Autodesk Fusion 360 part; units mm, degrees
note: some values were not read from the file. Chosen so that the rebuilt part matches the saved one: which bodies a step acts on.
(part 4 of 5)
sketch "スケッチ1 (16)" plane through (0, 0, 0) normal (0, 0, 1) x (1, 0, 0) in component "Stage2_Planet_Gear_C"
  line L0 (-42.7218, 3.2284) -> (-43.6623, 3.4671)
  line L1 (-43.6623, 3.4671) -> (-44.4838, 3.4839)
  line L2 (-44.4838, 3.4839) -> (-45.3401, 3.3351)
  line L3 (-45.3401, 3.3351) -> (-46.2134, 3.0621)
  line L4 (-46.2134, 3.0621) -> (-46.3661, 2.098)
  line L5 (-46.3661, 2.098) -> (-45.6199, 1.5685)
  line L6 (-45.6199, 1.5685) -> (-44.8515, 1.1623)
  line L7 (-44.8515, 1.1623) -> (-44.065, 0.9245)
  line L8 (-44.065, 0.9245) -> (-43.0967, 0.8608)
  line L9 (-43.0967, 0.8608) -> (-43.125, 0)
  line L10 (-43.125, 0) -> (-43.0967, -0.8608)
  line L11 (-43.0967, -0.8608) -> (-44.065, -0.9245)
  line L12 (-44.065, -0.9245) -> (-44.8515, -1.1623)
  line L13 (-44.8515, -1.1623) -> (-45.6199, -1.5685)
  line L14 (-45.6199, -1.5685) -> (-46.3661, -2.098)
  line L15 (-46.3661, -2.098) -> (-46.2134, -3.0621)
  line L16 (-46.2134, -3.0621) -> (-45.3401, -3.3351)
  line L17 (-45.3401, -3.3351) -> (-44.4838, -3.4839)
  line L18 (-44.4838, -3.4839) -> (-43.6623, -3.4671)
  line L19 (-43.6623, -3.4671) -> (-42.7218, -3.2284)
  line L20 (-42.7218, -3.2284) -> (-42.4826, -4.0558)
  line L21 (-42.4826, -4.0558) -> (-42.1897, -4.8658)
  line L22 (-42.1897, -4.8658) -> (-43.091, -5.2256)
  line L23 (-43.091, -5.2256) -> (-43.7654, -5.6948)
  line L24 (-43.7654, -5.6948) -> (-44.3707, -6.3185)
  line L25 (-44.3707, -6.3185) -> (-44.9168, -7.0527)
  line L26 (-44.9168, -7.0527) -> (-44.4736, -7.9225)
  line L27 (-44.4736, -7.9225) -> (-43.5587, -7.9123)
  line L28 (-43.5587, -7.9123) -> (-42.6983, -7.7891)
  line L29 (-42.6983, -7.7891) -> (-41.9223, -7.5193)
  line L30 (-41.9223, -7.5193) -> (-41.1015, -7.0016)
  line L31 (-41.1015, -7.0016) -> (-40.6183, -7.7147)
  line L32 (-40.6183, -7.7147) -> (-40.0895, -8.3945)
  line L33 (-40.0895, -8.3945) -> (-40.8355, -9.0152)
  line L34 (-40.8355, -9.0152) -> (-41.3319, -9.6699)
  line L35 (-41.3319, -9.6699) -> (-41.7149, -10.4501)
  line L36 (-41.7149, -10.4501) -> (-42.0073, -11.317)
  line L37 (-42.0073, -11.317) -> (-41.317, -12.0073)
  line L38 (-41.317, -12.0073) -> (-40.4501, -11.7149)
  line L39 (-40.4501, -11.7149) -> (-39.6699, -11.3319)
  line L40 (-39.6699, -11.3319) -> (-39.0152, -10.8355)
  line L41 (-39.0152, -10.8355) -> (-38.3945, -10.0895)
  line L42 (-38.3945, -10.0895) -> (-37.7147, -10.6183)
  line L43 (-37.7147, -10.6183) -> (-37.0016, -11.1015)
  line L44 (-37.0016, -11.1015) -> (-37.5193, -11.9223)
  line L45 (-37.5193, -11.9223) -> (-37.7891, -12.6983)
  line L46 (-37.7891, -12.6983) -> (-37.9123, -13.5587)
  line L47 (-37.9123, -13.5587) -> (-37.9225, -14.4736)
  line L48 (-37.9225, -14.4736) -> (-37.0527, -14.9168)
  line L49 (-37.0527, -14.9168) -> (-36.3185, -14.3707)
  line L50 (-36.3185, -14.3707) -> (-35.6948, -13.7654)
  line L51 (-35.6948, -13.7654) -> (-35.2256, -13.091)
  line L52 (-35.2256, -13.091) -> (-34.8658, -12.1897)
  line L53 (-34.8658, -12.1897) -> (-34.0558, -12.4826)
  line L54 (-34.0558, -12.4826) -> (-33.2284, -12.7218)
  line L55 (-33.2284, -12.7218) -> (-33.4671, -13.6623)
  line L56 (-33.4671, -13.6623) -> (-33.4839, -14.4838)
  line L57 (-33.4839, -14.4838) -> (-33.3351, -15.3401)
  line L58 (-33.3351, -15.3401) -> (-33.0621, -16.2134)
  line L59 (-33.0621, -16.2134) -> (-32.098, -16.3661)
  line L60 (-32.098, -16.3661) -> (-31.5685, -15.6199)
  line L61 (-31.5685, -15.6199) -> (-31.1623, -14.8515)
  line L62 (-31.1623, -14.8515) -> (-30.9245, -14.065)
  line L63 (-30.9245, -14.065) -> (-30.8608, -13.0967)
  line L64 (-30.8608, -13.0967) -> (-30, -13.125)
  line L65 (-30, -13.125) -> (-29.1392, -13.0967)
  line L66 (-29.1392, -13.0967) -> (-29.0755, -14.065)
  line L67 (-29.0755, -14.065) -> (-28.8377, -14.8515)
  line L68 (-28.8377, -14.8515) -> (-28.4315, -15.6199)
  line L69 (-28.4315, -15.6199) -> (-27.902, -16.3661)
  line L70 (-27.902, -16.3661) -> (-26.9379, -16.2134)
  line L71 (-26.9379, -16.2134) -> (-26.6649, -15.3401)
  line L72 (-26.6649, -15.3401) -> (-26.5161, -14.4838)
  line L73 (-26.5161, -14.4838) -> (-26.5329, -13.6623)
  line L74 (-26.5329, -13.6623) -> (-26.7716, -12.7218)
  line L75 (-26.7716, -12.7218) -> (-25.9442, -12.4826)
  line L76 (-25.9442, -12.4826) -> (-25.1342, -12.1897)
  line L77 (-25.1342, -12.1897) -> (-24.7744, -13.091)
  line L78 (-24.7744, -13.091) -> (-24.3052, -13.7654)
  line L79 (-24.3052, -13.7654) -> (-23.6815, -14.3707)
  line L80 (-23.6815, -14.3707) -> (-22.9473, -14.9168)
  line L81 (-22.9473, -14.9168) -> (-22.0775, -14.4736)
  line L82 (-22.0775, -14.4736) -> (-22.0877, -13.5587)
  line L83 (-22.0877, -13.5587) -> (-22.2109, -12.6983)
  line L84 (-22.2109, -12.6983) -> (-22.4807, -11.9223)
  line L85 (-22.4807, -11.9223) -> (-22.9984, -11.1015)
  line L86 (-22.9984, -11.1015) -> (-22.2853, -10.6183)
  line L87 (-22.2853, -10.6183) -> (-21.6055, -10.0895)
  line L88 (-21.6055, -10.0895) -> (-20.9848, -10.8355)
  line L89 (-20.9848, -10.8355) -> (-20.3301, -11.3319)
  line L90 (-20.3301, -11.3319) -> (-19.5499, -11.7149)
  line L91 (-19.5499, -11.7149) -> (-18.683, -12.0073)
  line L92 (-18.683, -12.0073) -> (-17.9927, -11.317)
  line L93 (-17.9927, -11.317) -> (-18.2851, -10.4501)
  line L94 (-18.2851, -10.4501) -> (-18.6681, -9.6699)
  line L95 (-18.6681, -9.6699) -> (-19.1645, -9.0152)
  line L96 (-19.1645, -9.0152) -> (-19.9105, -8.3945)
  line L97 (-19.9105, -8.3945) -> (-19.3817, -7.7147)
  line L98 (-19.3817, -7.7147) -> (-18.8985, -7.0016)
  line L99 (-18.8985, -7.0016) -> (-18.0777, -7.5193)
  line L100 (-18.0777, -7.5193) -> (-17.3017, -7.7891)
  line L101 (-17.3017, -7.7891) -> (-16.4413, -7.9123)
  line L102 (-16.4413, -7.9123) -> (-15.5264, -7.9225)
  line L103 (-15.5264, -7.9225) -> (-15.0832, -7.0527)
  line L104 (-15.0832, -7.0527) -> (-15.6293, -6.3185)
  line L105 (-15.6293, -6.3185) -> (-16.2346, -5.6948)
  line L106 (-16.2346, -5.6948) -> (-16.909, -5.2256)
  line L107 (-16.909, -5.2256) -> (-17.8103, -4.8658)
  line L108 (-17.8103, -4.8658) -> (-17.5174, -4.0558)
  line L109 (-17.5174, -4.0558) -> (-17.2782, -3.2284)
  line L110 (-17.2782, -3.2284) -> (-16.3377, -3.4671)
  line L111 (-16.3377, -3.4671) -> (-15.5162, -3.4839)
  line L112 (-15.5162, -3.4839) -> (-14.6599, -3.3351)
  line L113 (-14.6599, -3.3351) -> (-13.7866, -3.0621)
  line L114 (-13.7866, -3.0621) -> (-13.6339, -2.098)
  line L115 (-13.6339, -2.098) -> (-14.3801, -1.5685)
  line L116 (-14.3801, -1.5685) -> (-15.1485, -1.1623)
  line L117 (-15.1485, -1.1623) -> (-15.935, -0.9245)
  line L118 (-15.935, -0.9245) -> (-16.9033, -0.8608)
  line L119 (-16.9033, -0.8608) -> (-16.875, 0)
  line L120 (-16.875, 0) -> (-16.9033, 0.8608)
  line L121 (-16.9033, 0.8608) -> (-15.935, 0.9245)
  line L122 (-15.935, 0.9245) -> (-15.1485, 1.1623)
  line L123 (-15.1485, 1.1623) -> (-14.3801, 1.5685)
  line L124 (-14.3801, 1.5685) -> (-13.6339, 2.098)
  line L125 (-13.6339, 2.098) -> (-13.7866, 3.0621)
  line L126 (-13.7866, 3.0621) -> (-14.6599, 3.3351)
  line L127 (-14.6599, 3.3351) -> (-15.5162, 3.4839)
  line L128 (-15.5162, 3.4839) -> (-16.3377, 3.4671)
  line L129 (-16.3377, 3.4671) -> (-17.2782, 3.2284)
  line L130 (-17.2782, 3.2284) -> (-17.5174, 4.0558)
  line L131 (-17.5174, 4.0558) -> (-17.8103, 4.8658)
  line L132 (-17.8103, 4.8658) -> (-16.909, 5.2256)
  line L133 (-16.909, 5.2256) -> (-16.2346, 5.6948)
  line L134 (-16.2346, 5.6948) -> (-15.6293, 6.3185)
  line L135 (-15.6293, 6.3185) -> (-15.0832, 7.0527)
  line L136 (-15.0832, 7.0527) -> (-15.5264, 7.9225)
  line L137 (-15.5264, 7.9225) -> (-16.4413, 7.9123)
  line L138 (-16.4413, 7.9123) -> (-17.3017, 7.7891)
  line L139 (-17.3017, 7.7891) -> (-18.0777, 7.5193)
  line L140 (-18.0777, 7.5193) -> (-18.8985, 7.0016)
  line L141 (-18.8985, 7.0016) -> (-19.3817, 7.7147)
  line L142 (-19.3817, 7.7147) -> (-19.9105, 8.3945)
  line L143 (-19.9105, 8.3945) -> (-19.1645, 9.0152)
  line L144 (-19.1645, 9.0152) -> (-18.6681, 9.6699)
  line L145 (-18.6681, 9.6699) -> (-18.2851, 10.4501)
  line L146 (-18.2851, 10.4501) -> (-17.9927, 11.317)
  line L147 (-17.9927, 11.317) -> (-18.683, 12.0073)
  line L148 (-18.683, 12.0073) -> (-19.5499, 11.7149)
  line L149 (-19.5499, 11.7149) -> (-20.3301, 11.3319)
  line L150 (-20.3301, 11.3319) -> (-20.9848, 10.8355)
  line L151 (-20.9848, 10.8355) -> (-21.6055, 10.0895)
  line L152 (-21.6055, 10.0895) -> (-22.2853, 10.6183)
  line L153 (-22.2853, 10.6183) -> (-22.9984, 11.1015)
  line L154 (-22.9984, 11.1015) -> (-22.4807, 11.9223)
  line L155 (-22.4807, 11.9223) -> (-22.2109, 12.6983)
  line L156 (-22.2109, 12.6983) -> (-22.0877, 13.5587)
  line L157 (-22.0877, 13.5587) -> (-22.0775, 14.4736)
  line L158 (-22.0775, 14.4736) -> (-22.9473, 14.9168)
  line L159 (-22.9473, 14.9168) -> (-23.6815, 14.3707)
  line L160 (-23.6815, 14.3707) -> (-24.3052, 13.7654)
  line L161 (-24.3052, 13.7654) -> (-24.7744, 13.091)
  line L162 (-24.7744, 13.091) -> (-25.1342, 12.1897)
  line L163 (-25.1342, 12.1897) -> (-25.9442, 12.4826)
  line L164 (-25.9442, 12.4826) -> (-26.7716, 12.7218)
  line L165 (-26.7716, 12.7218) -> (-26.5329, 13.6623)
  line L166 (-26.5329, 13.6623) -> (-26.5161, 14.4838)
  line L167 (-26.5161, 14.4838) -> (-26.6649, 15.3401)
  line L168 (-26.6649, 15.3401) -> (-26.9379, 16.2134)
  line L169 (-26.9379, 16.2134) -> (-27.902, 16.3661)
  line L170 (-27.902, 16.3661) -> (-28.4315, 15.6199)
  line L171 (-28.4315, 15.6199) -> (-28.8377, 14.8515)
  line L172 (-28.8377, 14.8515) -> (-29.0755, 14.065)
  line L173 (-29.0755, 14.065) -> (-29.1392, 13.0967)
  line L174 (-29.1392, 13.0967) -> (-30, 13.125)
  line L175 (-30, 13.125) -> (-30.8608, 13.0967)
  line L176 (-30.8608, 13.0967) -> (-30.9245, 14.065)
  line L177 (-30.9245, 14.065) -> (-31.1623, 14.8515)
  line L178 (-31.1623, 14.8515) -> (-31.5685, 15.6199)
  line L179 (-31.5685, 15.6199) -> (-32.098, 16.3661)
  line L180 (-32.098, 16.3661) -> (-33.0621, 16.2134)
  line L181 (-33.0621, 16.2134) -> (-33.3351, 15.3401)
  line L182 (-33.3351, 15.3401) -> (-33.4839, 14.4838)
  line L183 (-33.4839, 14.4838) -> (-33.4671, 13.6623)
  line L184 (-33.4671, 13.6623) -> (-33.2284, 12.7218)
  line L185 (-33.2284, 12.7218) -> (-34.0558, 12.4826)
  line L186 (-34.0558, 12.4826) -> (-34.8658, 12.1897)
  line L187 (-34.8658, 12.1897) -> (-35.2256, 13.091)
  line L188 (-35.2256, 13.091) -> (-35.6948, 13.7654)
  line L189 (-35.6948, 13.7654) -> (-36.3185, 14.3707)
  line L190 (-36.3185, 14.3707) -> (-37.0527, 14.9168)
  line L191 (-37.0527, 14.9168) -> (-37.9225, 14.4736)
  line L192 (-37.9225, 14.4736) -> (-37.9123, 13.5587)
  line L193 (-37.9123, 13.5587) -> (-37.7891, 12.6983)
  line L194 (-37.7891, 12.6983) -> (-37.5193, 11.9223)
  line L195 (-37.5193, 11.9223) -> (-37.0016, 11.1015)
  line L196 (-37.0016, 11.1015) -> (-37.7147, 10.6183)
  line L197 (-37.7147, 10.6183) -> (-38.3945, 10.0895)
  line L198 (-38.3945, 10.0895) -> (-39.0152, 10.8355)
  line L199 (-39.0152, 10.8355) -> (-39.6699, 11.3319)
  line L200 (-39.6699, 11.3319) -> (-40.4501, 11.7149)
  line L201 (-40.4501, 11.7149) -> (-41.317, 12.0073)
  line L202 (-41.317, 12.0073) -> (-42.0073, 11.317)
  line L203 (-42.0073, 11.317) -> (-41.7149, 10.4501)
  line L204 (-41.7149, 10.4501) -> (-41.3319, 9.6699)
  line L205 (-41.3319, 9.6699) -> (-40.8355, 9.0152)
  line L206 (-40.8355, 9.0152) -> (-40.0895, 8.3945)
  line L207 (-40.0895, 8.3945) -> (-40.6183, 7.7147)
  line L208 (-40.6183, 7.7147) -> (-41.1015, 7.0016)
  line L209 (-41.1015, 7.0016) -> (-41.9223, 7.5193)
  line L210 (-41.9223, 7.5193) -> (-42.6983, 7.7891)
  line L211 (-42.6983, 7.7891) -> (-43.5587, 7.9123)
  line L212 (-43.5587, 7.9123) -> (-44.4736, 7.9225)
  line L213 (-44.4736, 7.9225) -> (-44.9168, 7.0527)
  line L214 (-44.9168, 7.0527) -> (-44.3707, 6.3185)
  line L215 (-44.3707, 6.3185) -> (-43.7654, 5.6948)
  line L216 (-43.7654, 5.6948) -> (-43.091, 5.2256)
  line L217 (-43.091, 5.2256) -> (-42.1897, 4.8658)
  line L218 (-42.1897, 4.8658) -> (-42.4826, 4.0558)
  line L219 (-42.4826, 4.0558) -> (-42.7218, 3.2284)
extrude "Stage2_Planet_C_Extrude" add sketch "スケッチ1 (16)" along normal blind 12 from surface at 74 separate body makes body 17 in component "Stage2_Planet_Gear_C"
sketch "スケッチ2 (16)" plane through (0, 0, 0) normal (0, 0, 1) x (1, 0, 0) in component "Stage2_Planet_Gear_C"
  circle A0 centre (-30, 0) radius 9
extrude "Stage2_Planet_C_Hub_Lower_Extrude" add sketch "スケッチ2 (16)" along normal blind 3 from surface at 71 bodies 17 in component "Stage2_Planet_Gear_C"
sketch "スケッチ3 (15)" plane through (0, 0, 0) normal (0, 0, 1) x (1, 0, 0) in component "Stage2_Planet_Gear_C"
  circle A0 centre (-30, 0) radius 9
extrude "Stage2_Planet_C_Hub_Upper_Extrude" add sketch "スケッチ3 (15)" along normal blind 3 from surface at 86 bodies 17 in component "Stage2_Planet_Gear_C"
sketch "スケッチ4 (15)" plane through (0, 0, 0) normal (0, 0, 1) x (1, 0, 0) in component "Stage2_Planet_Gear_C"
  circle A0 centre (-30, 0) radius 4.3
extrude "Stage2_Planet_C_Bore_Cut" cut sketch "スケッチ4 (15)" along normal blind 20 from surface at 70 bodies 17 in component "Stage2_Planet_Gear_C"
sketch "スケッチ1 (17)" plane through (0, 0, 0) normal (0, 0, 1) x (1, 0, 0) in component "Stage2_Planet_Gear_D"
  line L0 (-12.7218, -26.7716) -> (-13.6623, -26.5329)
  line L1 (-13.6623, -26.5329) -> (-14.4838, -26.5161)
  line L2 (-14.4838, -26.5161) -> (-15.3401, -26.6649)
  line L3 (-15.3401, -26.6649) -> (-16.2134, -26.9379)
  line L4 (-16.2134, -26.9379) -> (-16.3661, -27.902)
  line L5 (-16.3661, -27.902) -> (-15.6199, -28.4315)
  line L6 (-15.6199, -28.4315) -> (-14.8515, -28.8377)
  line L7 (-14.8515, -28.8377) -> (-14.065, -29.0755)
  line L8 (-14.065, -29.0755) -> (-13.0967, -29.1392)
  line L9 (-13.0967, -29.1392) -> (-13.125, -30)
  line L10 (-13.125, -30) -> (-13.0967, -30.8608)
  line L11 (-13.0967, -30.8608) -> (-14.065, -30.9245)
  line L12 (-14.065, -30.9245) -> (-14.8515, -31.1623)
  line L13 (-14.8515, -31.1623) -> (-15.6199, -31.5685)
  line L14 (-15.6199, -31.5685) -> (-16.3661, -32.098)
  line L15 (-16.3661, -32.098) -> (-16.2134, -33.0621)
  line L16 (-16.2134, -33.0621) -> (-15.3401, -33.3351)
  line L17 (-15.3401, -33.3351) -> (-14.4838, -33.4839)
  line L18 (-14.4838, -33.4839) -> (-13.6623, -33.4671)
  line L19 (-13.6623, -33.4671) -> (-12.7218, -33.2284)
  line L20 (-12.7218, -33.2284) -> (-12.4826, -34.0558)
  line L21 (-12.4826, -34.0558) -> (-12.1897, -34.8658)
  line L22 (-12.1897, -34.8658) -> (-13.091, -35.2256)
  line L23 (-13.091, -35.2256) -> (-13.7654, -35.6948)
  line L24 (-13.7654, -35.6948) -> (-14.3707, -36.3185)
  line L25 (-14.3707, -36.3185) -> (-14.9168, -37.0527)
  line L26 (-14.9168, -37.0527) -> (-14.4736, -37.9225)
  line L27 (-14.4736, -37.9225) -> (-13.5587, -37.9123)
  line L28 (-13.5587, -37.9123) -> (-12.6983, -37.7891)
  line L29 (-12.6983, -37.7891) -> (-11.9223, -37.5193)
  line L30 (-11.9223, -37.5193) -> (-11.1015, -37.0016)
  line L31 (-11.1015, -37.0016) -> (-10.6183, -37.7147)
  line L32 (-10.6183, -37.7147) -> (-10.0895, -38.3945)
  line L33 (-10.0895, -38.3945) -> (-10.8355, -39.0152)
  line L34 (-10.8355, -39.0152) -> (-11.3319, -39.6699)
  line L35 (-11.3319, -39.6699) -> (-11.7149, -40.4501)
  line L36 (-11.7149, -40.4501) -> (-12.0073, -41.317)
  line L37 (-12.0073, -41.317) -> (-11.317, -42.0073)
  line L38 (-11.317, -42.0073) -> (-10.4501, -41.7149)
  line L39 (-10.4501, -41.7149) -> (-9.6699, -41.3319)
  line L40 (-9.6699, -41.3319) -> (-9.0152, -40.8355)
  line L41 (-9.0152, -40.8355) -> (-8.3945, -40.0895)
  line L42 (-8.3945, -40.0895) -> (-7.7147, -40.6183)
  line L43 (-7.7147, -40.6183) -> (-7.0016, -41.1015)
  line L44 (-7.0016, -41.1015) -> (-7.5193, -41.9223)
  line L45 (-7.5193, -41.9223) -> (-7.7891, -42.6983)
  line L46 (-7.7891, -42.6983) -> (-7.9123, -43.5587)
  line L47 (-7.9123, -43.5587) -> (-7.9225, -44.4736)
  line L48 (-7.9225, -44.4736) -> (-7.0527, -44.9168)
  line L49 (-7.0527, -44.9168) -> (-6.3185, -44.3707)
  line L50 (-6.3185, -44.3707) -> (-5.6948, -43.7654)
  line L51 (-5.6948, -43.7654) -> (-5.2256, -43.091)
  line L52 (-5.2256, -43.091) -> (-4.8658, -42.1897)
  line L53 (-4.8658, -42.1897) -> (-4.0558, -42.4826)
  line L54 (-4.0558, -42.4826) -> (-3.2284, -42.7218)
  line L55 (-3.2284, -42.7218) -> (-3.4671, -43.6623)
  line L56 (-3.4671, -43.6623) -> (-3.4839, -44.4838)
  line L57 (-3.4839, -44.4838) -> (-3.3351, -45.3401)
  line L58 (-3.3351, -45.3401) -> (-3.0621, -46.2134)
  line L59 (-3.0621, -46.2134) -> (-2.098, -46.3661)
  line L60 (-2.098, -46.3661) -> (-1.5685, -45.6199)
  line L61 (-1.5685, -45.6199) -> (-1.1623, -44.8515)
  line L62 (-1.1623, -44.8515) -> (-0.9245, -44.065)
  line L63 (-0.9245, -44.065) -> (-0.8608, -43.0967)
  line L64 (-0.8608, -43.0967) -> (0, -43.125)
  line L65 (0, -43.125) -> (0.8608, -43.0967)
  line L66 (0.8608, -43.0967) -> (0.9245, -44.065)
  line L67 (0.9245, -44.065) -> (1.1623, -44.8515)
  line L68 (1.1623, -44.8515) -> (1.5685, -45.6199)
  line L69 (1.5685, -45.6199) -> (2.098, -46.3661)
  line L70 (2.098, -46.3661) -> (3.0621, -46.2134)
  line L71 (3.0621, -46.2134) -> (3.3351, -45.3401)
  line L72 (3.3351, -45.3401) -> (3.4839, -44.4838)
  line L73 (3.4839, -44.4838) -> (3.4671, -43.6623)
  line L74 (3.4671, -43.6623) -> (3.2284, -42.7218)
  line L75 (3.2284, -42.7218) -> (4.0558, -42.4826)
  line L76 (4.0558, -42.4826) -> (4.8658, -42.1897)
  line L77 (4.8658, -42.1897) -> (5.2256, -43.091)
  line L78 (5.2256, -43.091) -> (5.6948, -43.7654)
  line L79 (5.6948, -43.7654) -> (6.3185, -44.3707)
  line L80 (6.3185, -44.3707) -> (7.0527, -44.9168)
  line L81 (7.0527, -44.9168) -> (7.9225, -44.4736)
  line L82 (7.9225, -44.4736) -> (7.9123, -43.5587)
  line L83 (7.9123, -43.5587) -> (7.7891, -42.6983)
  line L84 (7.7891, -42.6983) -> (7.5193, -41.9223)
  line L85 (7.5193, -41.9223) -> (7.0016, -41.1015)
  line L86 (7.0016, -41.1015) -> (7.7147, -40.6183)
  line L87 (7.7147, -40.6183) -> (8.3945, -40.0895)
  line L88 (8.3945, -40.0895) -> (9.0152, -40.8355)
  line L89 (9.0152, -40.8355) -> (9.6699, -41.3319)
  line L90 (9.6699, -41.3319) -> (10.4501, -41.7149)
  line L91 (10.4501, -41.7149) -> (11.317, -42.0073)
  line L92 (11.317, -42.0073) -> (12.0073, -41.317)
  line L93 (12.0073, -41.317) -> (11.7149, -40.4501)
  line L94 (11.7149, -40.4501) -> (11.3319, -39.6699)
  line L95 (11.3319, -39.6699) -> (10.8355, -39.0152)
  line L96 (10.8355, -39.0152) -> (10.0895, -38.3945)
  line L97 (10.0895, -38.3945) -> (10.6183, -37.7147)
  line L98 (10.6183, -37.7147) -> (11.1015, -37.0016)
  line L99 (11.1015, -37.0016) -> (11.9223, -37.5193)
  line L100 (11.9223, -37.5193) -> (12.6983, -37.7891)
  line L101 (12.6983, -37.7891) -> (13.5587, -37.9123)
  line L102 (13.5587, -37.9123) -> (14.4736, -37.9225)
  line L103 (14.4736, -37.9225) -> (14.9168, -37.0527)
  line L104 (14.9168, -37.0527) -> (14.3707, -36.3185)
  line L105 (14.3707, -36.3185) -> (13.7654, -35.6948)
  line L106 (13.7654, -35.6948) -> (13.091, -35.2256)
  line L107 (13.091, -35.2256) -> (12.1897, -34.8658)
  line L108 (12.1897, -34.8658) -> (12.4826, -34.0558)
  line L109 (12.4826, -34.0558) -> (12.7218, -33.2284)
  line L110 (12.7218, -33.2284) -> (13.6623, -33.4671)
  line L111 (13.6623, -33.4671) -> (14.4838, -33.4839)
  line L112 (14.4838, -33.4839) -> (15.3401, -33.3351)
  line L113 (15.3401, -33.3351) -> (16.2134, -33.0621)
  line L114 (16.2134, -33.0621) -> (16.3661, -32.098)
  line L115 (16.3661, -32.098) -> (15.6199, -31.5685)
  line L116 (15.6199, -31.5685) -> (14.8515, -31.1623)
  line L117 (14.8515, -31.1623) -> (14.065, -30.9245)
  line L118 (14.065, -30.9245) -> (13.0967, -30.8608)
  line L119 (13.0967, -30.8608) -> (13.125, -30)
  line L120 (13.125, -30) -> (13.0967, -29.1392)
  line L121 (13.0967, -29.1392) -> (14.065, -29.0755)
  line L122 (14.065, -29.0755) -> (14.8515, -28.8377)
  line L123 (14.8515, -28.8377) -> (15.6199, -28.4315)
  line L124 (15.6199, -28.4315) -> (16.3661, -27.902)
  line L125 (16.3661, -27.902) -> (16.2134, -26.9379)
  line L126 (16.2134, -26.9379) -> (15.3401, -26.6649)
  line L127 (15.3401, -26.6649) -> (14.4838, -26.5161)
  line L128 (14.4838, -26.5161) -> (13.6623, -26.5329)
  line L129 (13.6623, -26.5329) -> (12.7218, -26.7716)
  line L130 (12.7218, -26.7716) -> (12.4826, -25.9442)
  line L131 (12.4826, -25.9442) -> (12.1897, -25.1342)
  line L132 (12.1897, -25.1342) -> (13.091, -24.7744)
  line L133 (13.091, -24.7744) -> (13.7654, -24.3052)
  line L134 (13.7654, -24.3052) -> (14.3707, -23.6815)
  line L135 (14.3707, -23.6815) -> (14.9168, -22.9473)
  line L136 (14.9168, -22.9473) -> (14.4736, -22.0775)
  line L137 (14.4736, -22.0775) -> (13.5587, -22.0877)
  line L138 (13.5587, -22.0877) -> (12.6983, -22.2109)
  line L139 (12.6983, -22.2109) -> (11.9223, -22.4807)
  line L140 (11.9223, -22.4807) -> (11.1015, -22.9984)
  line L141 (11.1015, -22.9984) -> (10.6183, -22.2853)
  line L142 (10.6183, -22.2853) -> (10.0895, -21.6055)
  line L143 (10.0895, -21.6055) -> (10.8355, -20.9848)
  line L144 (10.8355, -20.9848) -> (11.3319, -20.3301)
  line L145 (11.3319, -20.3301) -> (11.7149, -19.5499)
  line L146 (11.7149, -19.5499) -> (12.0073, -18.683)
  line L147 (12.0073, -18.683) -> (11.317, -17.9927)
  line L148 (11.317, -17.9927) -> (10.4501, -18.2851)
  line L149 (10.4501, -18.2851) -> (9.6699, -18.6681)
  line L150 (9.6699, -18.6681) -> (9.0152, -19.1645)
  line L151 (9.0152, -19.1645) -> (8.3945, -19.9105)
  line L152 (8.3945, -19.9105) -> (7.7147, -19.3817)
  line L153 (7.7147, -19.3817) -> (7.0016, -18.8985)
  line L154 (7.0016, -18.8985) -> (7.5193, -18.0777)
  line L155 (7.5193, -18.0777) -> (7.7891, -17.3017)
  line L156 (7.7891, -17.3017) -> (7.9123, -16.4413)
  line L157 (7.9123, -16.4413) -> (7.9225, -15.5264)
  line L158 (7.9225, -15.5264) -> (7.0527, -15.0832)
  line L159 (7.0527, -15.0832) -> (6.3185, -15.6293)
  line L160 (6.3185, -15.6293) -> (5.6948, -16.2346)
  line L161 (5.6948, -16.2346) -> (5.2256, -16.909)
  line L162 (5.2256, -16.909) -> (4.8658, -17.8103)
  line L163 (4.8658, -17.8103) -> (4.0558, -17.5174)
  line L164 (4.0558, -17.5174) -> (3.2284, -17.2782)
  line L165 (3.2284, -17.2782) -> (3.4671, -16.3377)
  line L166 (3.4671, -16.3377) -> (3.4839, -15.5162)
  line L167 (3.4839, -15.5162) -> (3.3351, -14.6599)
  line L168 (3.3351, -14.6599) -> (3.0621, -13.7866)
  line L169 (3.0621, -13.7866) -> (2.098, -13.6339)
  line L170 (2.098, -13.6339) -> (1.5685, -14.3801)
  line L171 (1.5685, -14.3801) -> (1.1623, -15.1485)
  line L172 (1.1623, -15.1485) -> (0.9245, -15.935)
  line L173 (0.9245, -15.935) -> (0.8608, -16.9033)
  line L174 (0.8608, -16.9033) -> (0, -16.875)
  line L175 (0, -16.875) -> (-0.8608, -16.9033)
  line L176 (-0.8608, -16.9033) -> (-0.9245, -15.935)
  line L177 (-0.9245, -15.935) -> (-1.1623, -15.1485)
  line L178 (-1.1623, -15.1485) -> (-1.5685, -14.3801)
  line L179 (-1.5685, -14.3801) -> (-2.098, -13.6339)
  line L180 (-2.098, -13.6339) -> (-3.0621, -13.7866)
  line L181 (-3.0621, -13.7866) -> (-3.3351, -14.6599)
  line L182 (-3.3351, -14.6599) -> (-3.4839, -15.5162)
  line L183 (-3.4839, -15.5162) -> (-3.4671, -16.3377)
  line L184 (-3.4671, -16.3377) -> (-3.2284, -17.2782)
  line L185 (-3.2284, -17.2782) -> (-4.0558, -17.5174)
  line L186 (-4.0558, -17.5174) -> (-4.8658, -17.8103)
  line L187 (-4.8658, -17.8103) -> (-5.2256, -16.909)
  line L188 (-5.2256, -16.909) -> (-5.6948, -16.2346)
  line L189 (-5.6948, -16.2346) -> (-6.3185, -15.6293)
  line L190 (-6.3185, -15.6293) -> (-7.0527, -15.0832)
  line L191 (-7.0527, -15.0832) -> (-7.9225, -15.5264)
  line L192 (-7.9225, -15.5264) -> (-7.9123, -16.4413)
  line L193 (-7.9123, -16.4413) -> (-7.7891, -17.3017)
  line L194 (-7.7891, -17.3017) -> (-7.5193, -18.0777)
  line L195 (-7.5193, -18.0777) -> (-7.0016, -18.8985)
  line L196 (-7.0016, -18.8985) -> (-7.7147, -19.3817)
  line L197 (-7.7147, -19.3817) -> (-8.3945, -19.9105)
  line L198 (-8.3945, -19.9105) -> (-9.0152, -19.1645)
  line L199 (-9.0152, -19.1645) -> (-9.6699, -18.6681)
  line L200 (-9.6699, -18.6681) -> (-10.4501, -18.2851)
  line L201 (-10.4501, -18.2851) -> (-11.317, -17.9927)
  line L202 (-11.317, -17.9927) -> (-12.0073, -18.683)
  line L203 (-12.0073, -18.683) -> (-11.7149, -19.5499)
  line L204 (-11.7149, -19.5499) -> (-11.3319, -20.3301)
  line L205 (-11.3319, -20.3301) -> (-10.8355, -20.9848)
  line L206 (-10.8355, -20.9848) -> (-10.0895, -21.6055)
  line L207 (-10.0895, -21.6055) -> (-10.6183, -22.2853)
  line L208 (-10.6183, -22.2853) -> (-11.1015, -22.9984)
  line L209 (-11.1015, -22.9984) -> (-11.9223, -22.4807)
  line L210 (-11.9223, -22.4807) -> (-12.6983, -22.2109)
  line L211 (-12.6983, -22.2109) -> (-13.5587, -22.0877)
  line L212 (-13.5587, -22.0877) -> (-14.4736, -22.0775)
  line L213 (-14.4736, -22.0775) -> (-14.9168, -22.9473)
  line L214 (-14.9168, -22.9473) -> (-14.3707, -23.6815)
  line L215 (-14.3707, -23.6815) -> (-13.7654, -24.3052)
  line L216 (-13.7654, -24.3052) -> (-13.091, -24.7744)
  line L217 (-13.091, -24.7744) -> (-12.1897, -25.1342)
  line L218 (-12.1897, -25.1342) -> (-12.4826, -25.9442)
  line L219 (-12.4826, -25.9442) -> (-12.7218, -26.7716)
extrude "Stage2_Planet_D_Extrude" add sketch "スケッチ1 (17)" along normal blind 12 from surface at 74 separate body makes body 18 in component "Stage2_Planet_Gear_D"
sketch "スケッチ2 (17)" plane through (0, 0, 0) normal (0, 0, 1) x (1, 0, 0) in component "Stage2_Planet_Gear_D"
  circle A0 centre (0, -30) radius 9
extrude "Stage2_Planet_D_Hub_Lower_Extrude" add sketch "スケッチ2 (17)" along normal blind 3 from surface at 71 bodies 18 in component "Stage2_Planet_Gear_D"
sketch "スケッチ3 (16)" plane through (0, 0, 0) normal (0, 0, 1) x (1, 0, 0) in component "Stage2_Planet_Gear_D"
  circle A0 centre (0, -30) radius 9
extrude "Stage2_Planet_D_Hub_Upper_Extrude" add sketch "スケッチ3 (16)" along normal blind 3 from surface at 86 bodies 18 in component "Stage2_Planet_Gear_D"
sketch "スケッチ4 (16)" plane through (0, 0, 0) normal (0, 0, 1) x (1, 0, 0) in component "Stage2_Planet_Gear_D"
  circle A0 centre (0, -30) radius 4.3
extrude "Stage2_Planet_D_Bore_Cut" cut sketch "スケッチ4 (16)" along normal blind 20 from surface at 70 bodies 18 in component "Stage2_Planet_Gear_D"
sketch "スケッチ1 (18)" plane through (0, 0, 0) normal (0, 0, 1) x (1, 0, 0) in component "Stage2_Internal_Ring_Gear"
  circle A0 centre (0, 0) radius 58
extrude "Stage2_Ring_Extrude" add sketch "スケッチ1 (18)" along normal blind 12 from surface at 74 separate body makes body 19 in component "Stage2_Internal_Ring_Gear"
sketch "スケッチ2 (18)" plane through (0, 0, 0) normal (0, 0, 1) x (1, 0, 0) in component "Stage2_Internal_Ring_Gear"
  circle A0 centre (0, 0) radius 65.5
extrude "Stage2_Ring_Flange_Extrude" add sketch "スケッチ2 (18)" along normal blind 7 from surface at 76.5 bodies 19 in component "Stage2_Internal_Ring_Gear"
sketch "スケッチ3 (17)" plane through (0, 0, 0) normal (0, 0, 1) x (1, 0, 0) in component "Stage2_Internal_Ring_Gear"
  line L0 (46.8321, -2.0047) -> (45.171, -1.2223)
  line L1 (45.171, -1.2223) -> (43.495, -0.6584)
  line L2 (43.495, -0.6584) -> (43.495, 0.6584)
  line L3 (43.495, 0.6584) -> (45.171, 1.2223)
  line L4 (45.171, 1.2223) -> (46.8321, 2.0047)
  line L5 (46.8321, 2.0047) -> (46.8108, 2.4532)
  line L6 (46.8108, 2.4532) -> (46.7851, 2.9016)
  line L7 (46.7851, 2.9016) -> (45.0513, 3.506)
  line L8 (45.0513, 3.506) -> (43.3256, 3.8917)
  line L9 (43.3256, 3.8917) -> (43.1879, 5.2013)
  line L10 (43.1879, 5.2013) -> (44.7957, 5.9373)
  line L11 (44.7957, 5.9373) -> (46.366, 6.889)
  line L12 (46.366, 6.889) -> (46.2979, 7.3329)
  line L13 (46.2979, 7.3329) -> (46.2255, 7.7761)
  line L14 (46.2255, 7.7761) -> (44.438, 8.196)
  line L15 (44.438, 8.196) -> (42.6814, 8.3991)
  line L16 (42.6814, 8.3991) -> (42.4077, 9.6871)
  line L17 (42.4077, 9.6871) -> (43.9297, 10.5872)
  line L18 (43.9297, 10.5872) -> (45.3919, 11.6978)
  line L19 (45.3919, 11.6978) -> (45.2778, 12.1321)
  line L20 (45.2778, 12.1321) -> (45.1595, 12.5653)
  line L21 (45.1595, 12.5653) -> (43.3379, 12.7961)
  line L22 (43.3379, 12.7961) -> (41.5697, 12.8145)
  line L23 (41.5697, 12.8145) -> (41.1628, 14.0669)
  line L24 (41.1628, 14.0669) -> (42.5824, 15.1211)
  line L25 (42.5824, 15.1211) -> (43.9205, 16.3785)
  line L26 (43.9205, 16.3785) -> (43.7616, 16.7985)
  line L27 (43.7616, 16.7985) -> (43.5986, 17.217)
  line L28 (43.5986, 17.217) -> (41.7629, 17.256)
  line L29 (41.7629, 17.256) -> (40.0025, 17.0895)
  line L30 (40.0025, 17.0895) -> (39.4669, 18.2925)
  line L31 (39.4669, 18.2925) -> (40.7686, 19.4893)
  line L32 (40.7686, 19.4893) -> (41.9679, 20.8797)
  line L33 (41.9679, 20.8797) -> (41.7659, 21.2808)
  line L34 (41.7659, 21.2808) -> (41.5601, 21.6799)
  line L35 (41.5601, 21.6799) -> (39.7304, 21.5269)
  line L36 (39.7304, 21.5269) -> (37.997, 21.1773)
  line L37 (37.997, 21.1773) -> (37.3386, 22.3177)
  line L38 (37.3386, 22.3177) -> (38.508, 23.644)
  line L39 (38.508, 23.644) -> (39.5555, 25.1522)
  line L40 (39.5555, 25.1522) -> (39.3127, 25.53)
  line L41 (39.3127, 25.53) -> (39.0663, 25.9054)
  line L42 (39.0663, 25.9054) -> (37.2625, 25.5619)
  line L43 (37.2625, 25.5619) -> (35.5752, 25.0331)
  line L44 (35.5752, 25.0331) -> (34.8012, 26.0984)
  line L45 (34.8012, 26.0984) -> (35.8256, 27.5397)
  line L46 (35.8256, 27.5397) -> (36.7096, 29.1491)
  line L47 (36.7096, 29.1491) -> (36.4287, 29.4994)
  line L48 (36.4287, 29.4994) -> (36.1444, 29.847)
  line L49 (36.1444, 29.847) -> (34.3865, 29.3169)
  line L50 (34.3865, 29.3169) -> (32.7636, 28.6146)
  line L51 (32.7636, 28.6146) -> (31.8825, 29.5931)
  line L52 (31.8825, 29.5931) -> (32.7507, 31.1336)
  line L53 (32.7507, 31.1336) -> (33.4616, 32.8266)
  line L54 (33.4616, 32.8266) -> (33.1456, 33.1456)
  line L55 (33.1456, 33.1456) -> (32.8266, 33.4616)
  line L56 (32.8266, 33.4616) -> (31.1336, 32.7507)
  line L57 (31.1336, 32.7507) -> (29.5931, 31.8825)
  line L58 (29.5931, 31.8825) -> (28.6146, 32.7636)
  line L59 (28.6146, 32.7636) -> (29.3169, 34.3865)
  line L60 (29.3169, 34.3865) -> (29.847, 36.1444)
  line L61 (29.847, 36.1444) -> (29.4994, 36.4287)
  line L62 (29.4994, 36.4287) -> (29.1491, 36.7096)
  line L63 (29.1491, 36.7096) -> (27.5397, 35.8256)
  line L64 (27.5397, 35.8256) -> (26.0984, 34.8012)
  line L65 (26.0984, 34.8012) -> (25.0331, 35.5752)
  line L66 (25.0331, 35.5752) -> (25.5619, 37.2625)
  line L67 (25.5619, 37.2625) -> (25.9054, 39.0663)
  line L68 (25.9054, 39.0663) -> (25.53, 39.3127)
  line L69 (25.53, 39.3127) -> (25.1522, 39.5555)
  line L70 (25.1522, 39.5555) -> (23.644, 38.508)
  line L71 (23.644, 38.508) -> (22.3177, 37.3386)
  line L72 (22.3177, 37.3386) -> (21.1773, 37.997)
  line L73 (21.1773, 37.997) -> (21.5269, 39.7304)
  line L74 (21.5269, 39.7304) -> (21.6799, 41.5601)
  line L75 (21.6799, 41.5601) -> (21.2808, 41.7659)
  line L76 (21.2808, 41.7659) -> (20.8797, 41.9679)
  line L77 (20.8797, 41.9679) -> (19.4893, 40.7686)
  line L78 (19.4893, 40.7686) -> (18.2925, 39.4669)
  line L79 (18.2925, 39.4669) -> (17.0895, 40.0025)
  line L80 (17.0895, 40.0025) -> (17.256, 41.7629)
  line L81 (17.256, 41.7629) -> (17.217, 43.5986)
  line L82 (17.217, 43.5986) -> (16.7985, 43.7616)
  line L83 (16.7985, 43.7616) -> (16.3785, 43.9205)
  line L84 (16.3785, 43.9205) -> (15.1211, 42.5824)
  line L85 (15.1211, 42.5824) -> (14.0669, 41.1628)
  line L86 (14.0669, 41.1628) -> (12.8145, 41.5697)
  line L87 (12.8145, 41.5697) -> (12.7961, 43.3379)
  line L88 (12.7961, 43.3379) -> (12.5653, 45.1595)
  line L89 (12.5653, 45.1595) -> (12.1321, 45.2778)
  line L90 (12.1321, 45.2778) -> (11.6978, 45.3919)
  line L91 (11.6978, 45.3919) -> (10.5872, 43.9297)
  line L92 (10.5872, 43.9297) -> (9.6871, 42.4077)
  line L93 (9.6871, 42.4077) -> (8.3991, 42.6814)
  line L94 (8.3991, 42.6814) -> (8.196, 44.438)
  line L95 (8.196, 44.438) -> (7.7761, 46.2255)
  line L96 (7.7761, 46.2255) -> (7.3329, 46.2979)
  line L97 (7.3329, 46.2979) -> (6.889, 46.366)
  line L98 (6.889, 46.366) -> (5.9373, 44.7957)
  line L99 (5.9373, 44.7957) -> (5.2013, 43.1879)
  line L100 (5.2013, 43.1879) -> (3.8917, 43.3256)
  line L101 (3.8917, 43.3256) -> (3.506, 45.0513)
  line L102 (3.506, 45.0513) -> (2.9016, 46.7851)
  line L103 (2.9016, 46.7851) -> (2.4532, 46.8108)
  line L104 (2.4532, 46.8108) -> (2.0047, 46.8321)
  line L105 (2.0047, 46.8321) -> (1.2223, 45.171)
  line L106 (1.2223, 45.171) -> (0.6584, 43.495)
  line L107 (0.6584, 43.495) -> (-0.6584, 43.495)
  line L108 (-0.6584, 43.495) -> (-1.2223, 45.171)
  line L109 (-1.2223, 45.171) -> (-2.0047, 46.8321)
  line L110 (-2.0047, 46.8321) -> (-2.4532, 46.8108)
  line L111 (-2.4532, 46.8108) -> (-2.9016, 46.7851)
  line L112 (-2.9016, 46.7851) -> (-3.506, 45.0513)
  line L113 (-3.506, 45.0513) -> (-3.8917, 43.3256)
  line L114 (-3.8917, 43.3256) -> (-5.2013, 43.1879)
  line L115 (-5.2013, 43.1879) -> (-5.9373, 44.7957)
  line L116 (-5.9373, 44.7957) -> (-6.889, 46.366)
  line L117 (-6.889, 46.366) -> (-7.3329, 46.2979)
  line L118 (-7.3329, 46.2979) -> (-7.7761, 46.2255)
  line L119 (-7.7761, 46.2255) -> (-8.196, 44.438)
  line L120 (-8.196, 44.438) -> (-8.3991, 42.6814)
  line L121 (-8.3991, 42.6814) -> (-9.6871, 42.4077)
  line L122 (-9.6871, 42.4077) -> (-10.5872, 43.9297)
  line L123 (-10.5872, 43.9297) -> (-11.6978, 45.3919)
  line L124 (-11.6978, 45.3919) -> (-12.1321, 45.2778)
  line L125 (-12.1321, 45.2778) -> (-12.5653, 45.1595)
  line L126 (-12.5653, 45.1595) -> (-12.7961, 43.3379)
  line L127 (-12.7961, 43.3379) -> (-12.8145, 41.5697)
  line L128 (-12.8145, 41.5697) -> (-14.0669, 41.1628)
  line L129 (-14.0669, 41.1628) -> (-15.1211, 42.5824)
  line L130 (-15.1211, 42.5824) -> (-16.3785, 43.9205)
  line L131 (-16.3785, 43.9205) -> (-16.7985, 43.7616)
  line L132 (-16.7985, 43.7616) -> (-17.217, 43.5986)
  line L133 (-17.217, 43.5986) -> (-17.256, 41.7629)
  line L134 (-17.256, 41.7629) -> (-17.0895, 40.0025)
  line L135 (-17.0895, 40.0025) -> (-18.2925, 39.4669)
  line L136 (-18.2925, 39.4669) -> (-19.4893, 40.7686)
  line L137 (-19.4893, 40.7686) -> (-20.8797, 41.9679)
  line L138 (-20.8797, 41.9679) -> (-21.2808, 41.7659)
  line L139 (-21.2808, 41.7659) -> (-21.6799, 41.5601)
  line L140 (-21.6799, 41.5601) -> (-21.5269, 39.7304)
  line L141 (-21.5269, 39.7304) -> (-21.1773, 37.997)
  line L142 (-21.1773, 37.997) -> (-22.3177, 37.3386)
  line L143 (-22.3177, 37.3386) -> (-23.644, 38.508)
  line L144 (-23.644, 38.508) -> (-25.1522, 39.5555)
  line L145 (-25.1522, 39.5555) -> (-25.53, 39.3127)
  line L146 (-25.53, 39.3127) -> (-25.9054, 39.0663)
  line L147 (-25.9054, 39.0663) -> (-25.5619, 37.2625)
  line L148 (-25.5619, 37.2625) -> (-25.0331, 35.5752)
  line L149 (-25.0331, 35.5752) -> (-26.0984, 34.8012)
  line L150 (-26.0984, 34.8012) -> (-27.5397, 35.8256)
  line L151 (-27.5397, 35.8256) -> (-29.1491, 36.7096)
  line L152 (-29.1491, 36.7096) -> (-29.4994, 36.4287)
  line L153 (-29.4994, 36.4287) -> (-29.847, 36.1444)
  line L154 (-29.847, 36.1444) -> (-29.3169, 34.3865)
  line L155 (-29.3169, 34.3865) -> (-28.6146, 32.7636)
  line L156 (-28.6146, 32.7636) -> (-29.5931, 31.8825)
  line L157 (-29.5931, 31.8825) -> (-31.1336, 32.7507)
  line L158 (-31.1336, 32.7507) -> (-32.8266, 33.4616)
  line L159 (-32.8266, 33.4616) -> (-33.1456, 33.1456)
  line L160 (-33.1456, 33.1456) -> (-33.4616, 32.8266)
  line L161 (-33.4616, 32.8266) -> (-32.7507, 31.1336)
  line L162 (-32.7507, 31.1336) -> (-31.8825, 29.5931)
  line L163 (-31.8825, 29.5931) -> (-32.7636, 28.6146)
  line L164 (-32.7636, 28.6146) -> (-34.3865, 29.3169)
  line L165 (-34.3865, 29.3169) -> (-36.1444, 29.847)
  line L166 (-36.1444, 29.847) -> (-36.4287, 29.4994)
  line L167 (-36.4287, 29.4994) -> (-36.7096, 29.1491)
  line L168 (-36.7096, 29.1491) -> (-35.8256, 27.5397)
  line L169 (-35.8256, 27.5397) -> (-34.8012, 26.0984)
  line L170 (-34.8012, 26.0984) -> (-35.5752, 25.0331)
  line L171 (-35.5752, 25.0331) -> (-37.2625, 25.5619)
  line L172 (-37.2625, 25.5619) -> (-39.0663, 25.9054)
  line L173 (-39.0663, 25.9054) -> (-39.3127, 25.53)
  line L174 (-39.3127, 25.53) -> (-39.5555, 25.1522)
  line L175 (-39.5555, 25.1522) -> (-38.508, 23.644)
  line L176 (-38.508, 23.644) -> (-37.3386, 22.3177)
  line L177 (-37.3386, 22.3177) -> (-37.997, 21.1773)
  line L178 (-37.997, 21.1773) -> (-39.7304, 21.5269)
  line L179 (-39.7304, 21.5269) -> (-41.5601, 21.6799)
  line L180 (-41.5601, 21.6799) -> (-41.7659, 21.2808)
  line L181 (-41.7659, 21.2808) -> (-41.9679, 20.8797)
  line L182 (-41.9679, 20.8797) -> (-40.7686, 19.4893)
  line L183 (-40.7686, 19.4893) -> (-39.4669, 18.2925)
  line L184 (-39.4669, 18.2925) -> (-40.0025, 17.0895)
  line L185 (-40.0025, 17.0895) -> (-41.7629, 17.256)
  line L186 (-41.7629, 17.256) -> (-43.5986, 17.217)
  line L187 (-43.5986, 17.217) -> (-43.7616, 16.7985)
  line L188 (-43.7616, 16.7985) -> (-43.9205, 16.3785)
  line L189 (-43.9205, 16.3785) -> (-42.5824, 15.1211)
  line L190 (-42.5824, 15.1211) -> (-41.1628, 14.0669)
  line L191 (-41.1628, 14.0669) -> (-41.5697, 12.8145)
  line L192 (-41.5697, 12.8145) -> (-43.3379, 12.7961)
  line L193 (-43.3379, 12.7961) -> (-45.1595, 12.5653)
  line L194 (-45.1595, 12.5653) -> (-45.2778, 12.1321)
  line L195 (-45.2778, 12.1321) -> (-45.3919, 11.6978)
  line L196 (-45.3919, 11.6978) -> (-43.9297, 10.5872)
  line L197 (-43.9297, 10.5872) -> (-42.4077, 9.6871)
  line L198 (-42.4077, 9.6871) -> (-42.6814, 8.3991)
  line L199 (-42.6814, 8.3991) -> (-44.438, 8.196)
  line L200 (-44.438, 8.196) -> (-46.2255, 7.7761)
  line L201 (-46.2255, 7.7761) -> (-46.2979, 7.3329)
  line L202 (-46.2979, 7.3329) -> (-46.366, 6.889)
  line L203 (-46.366, 6.889) -> (-44.7957, 5.9373)
  line L204 (-44.7957, 5.9373) -> (-43.1879, 5.2013)
  line L205 (-43.1879, 5.2013) -> (-43.3256, 3.8917)
  line L206 (-43.3256, 3.8917) -> (-45.0513, 3.506)
  line L207 (-45.0513, 3.506) -> (-46.7851, 2.9016)
  line L208 (-46.7851, 2.9016) -> (-46.8108, 2.4532)
  line L209 (-46.8108, 2.4532) -> (-46.8321, 2.0047)
  line L210 (-46.8321, 2.0047) -> (-45.171, 1.2223)
  line L211 (-45.171, 1.2223) -> (-43.495, 0.6584)
  line L212 (-43.495, 0.6584) -> (-43.495, -0.6584)
  line L213 (-43.495, -0.6584) -> (-45.171, -1.2223)
  line L214 (-45.171, -1.2223) -> (-46.8321, -2.0047)
  line L215 (-46.8321, -2.0047) -> (-46.8108, -2.4532)
  line L216 (-46.8108, -2.4532) -> (-46.7851, -2.9016)
  line L217 (-46.7851, -2.9016) -> (-45.0513, -3.506)
  line L218 (-45.0513, -3.506) -> (-43.3256, -3.8917)
  line L219 (-43.3256, -3.8917) -> (-43.1879, -5.2013)
  line L220 (-43.1879, -5.2013) -> (-44.7957, -5.9373)
  line L221 (-44.7957, -5.9373) -> (-46.366, -6.889)
  line L222 (-46.366, -6.889) -> (-46.2979, -7.3329)
  line L223 (-46.2979, -7.3329) -> (-46.2255, -7.7761)
  line L224 (-46.2255, -7.7761) -> (-44.438, -8.196)
  line L225 (-44.438, -8.196) -> (-42.6814, -8.3991)
  line L226 (-42.6814, -8.3991) -> (-42.4077, -9.6871)
  line L227 (-42.4077, -9.6871) -> (-43.9297, -10.5872)
  line L228 (-43.9297, -10.5872) -> (-45.3919, -11.6978)
  line L229 (-45.3919, -11.6978) -> (-45.2778, -12.1321)
  line L230 (-45.2778, -12.1321) -> (-45.1595, -12.5653)
  line L231 (-45.1595, -12.5653) -> (-43.3379, -12.7961)
  line L232 (-43.3379, -12.7961) -> (-41.5697, -12.8145)
  line L233 (-41.5697, -12.8145) -> (-41.1628, -14.0669)
  line L234 (-41.1628, -14.0669) -> (-42.5824, -15.1211)
  line L235 (-42.5824, -15.1211) -> (-43.9205, -16.3785)
  line L236 (-43.9205, -16.3785) -> (-43.7616, -16.7985)
  line L237 (-43.7616, -16.7985) -> (-43.5986, -17.217)
  line L238 (-43.5986, -17.217) -> (-41.7629, -17.256)
  line L239 (-41.7629, -17.256) -> (-40.0025, -17.0895)
  line L240 (-40.0025, -17.0895) -> (-39.4669, -18.2925)
  line L241 (-39.4669, -18.2925) -> (-40.7686, -19.4893)
  line L242 (-40.7686, -19.4893) -> (-41.9679, -20.8797)
  line L243 (-41.9679, -20.8797) -> (-41.7659, -21.2808)
  line L244 (-41.7659, -21.2808) -> (-41.5601, -21.6799)
  line L245 (-41.5601, -21.6799) -> (-39.7304, -21.5269)
  line L246 (-39.7304, -21.5269) -> (-37.997, -21.1773)
  line L247 (-37.997, -21.1773) -> (-37.3386, -22.3177)
  line L248 (-37.3386, -22.3177) -> (-38.508, -23.644)
  line L249 (-38.508, -23.644) -> (-39.5555, -25.1522)
  line L250 (-39.5555, -25.1522) -> (-39.3127, -25.53)
  line L251 (-39.3127, -25.53) -> (-39.0663, -25.9054)
  line L252 (-39.0663, -25.9054) -> (-37.2625, -25.5619)
  line L253 (-37.2625, -25.5619) -> (-35.5752, -25.0331)
  line L254 (-35.5752, -25.0331) -> (-34.8012, -26.0984)
  line L255 (-34.8012, -26.0984) -> (-35.8256, -27.5397)
  line L256 (-35.8256, -27.5397) -> (-36.7096, -29.1491)
  line L257 (-36.7096, -29.1491) -> (-36.4287, -29.4994)
  line L258 (-36.4287, -29.4994) -> (-36.1444, -29.847)
  line L259 (-36.1444, -29.847) -> (-34.3865, -29.3169)
  line L260 (-34.3865, -29.3169) -> (-32.7636, -28.6146)
  line L261 (-32.7636, -28.6146) -> (-31.8825, -29.5931)
  line L262 (-31.8825, -29.5931) -> (-32.7507, -31.1336)
  line L263 (-32.7507, -31.1336) -> (-33.4616, -32.8266)
  line L264 (-33.4616, -32.8266) -> (-33.1456, -33.1456)
  line L265 (-33.1456, -33.1456) -> (-32.8266, -33.4616)
  line L266 (-32.8266, -33.4616) -> (-31.1336, -32.7507)
  line L267 (-31.1336, -32.7507) -> (-29.5931, -31.8825)
  line L268 (-29.5931, -31.8825) -> (-28.6146, -32.7636)
  line L269 (-28.6146, -32.7636) -> (-29.3169, -34.3865)
  line L270 (-29.3169, -34.3865) -> (-29.847, -36.1444)
  line L271 (-29.847, -36.1444) -> (-29.4994, -36.4287)
  line L272 (-29.4994, -36.4287) -> (-29.1491, -36.7096)
  line L273 (-29.1491, -36.7096) -> (-27.5397, -35.8256)
  line L274 (-27.5397, -35.8256) -> (-26.0984, -34.8012)
  line L275 (-26.0984, -34.8012) -> (-25.0331, -35.5752)
  line L276 (-25.0331, -35.5752) -> (-25.5619, -37.2625)
  line L277 (-25.5619, -37.2625) -> (-25.9054, -39.0663)
  line L278 (-25.9054, -39.0663) -> (-25.53, -39.3127)
  line L279 (-25.53, -39.3127) -> (-25.1522, -39.5555)
  line L280 (-25.1522, -39.5555) -> (-23.644, -38.508)
  line L281 (-23.644, -38.508) -> (-22.3177, -37.3386)
  line L282 (-22.3177, -37.3386) -> (-21.1773, -37.997)
  line L283 (-21.1773, -37.997) -> (-21.5269, -39.7304)
  line L284 (-21.5269, -39.7304) -> (-21.6799, -41.5601)
  line L285 (-21.6799, -41.5601) -> (-21.2808, -41.7659)
  line L286 (-21.2808, -41.7659) -> (-20.8797, -41.9679)
  line L287 (-20.8797, -41.9679) -> (-19.4893, -40.7686)
  line L288 (-19.4893, -40.7686) -> (-18.2925, -39.4669)
  line L289 (-18.2925, -39.4669) -> (-17.0895, -40.0025)
  line L290 (-17.0895, -40.0025) -> (-17.256, -41.7629)
  line L291 (-17.256, -41.7629) -> (-17.217, -43.5986)
  line L292 (-17.217, -43.5986) -> (-16.7985, -43.7616)
  line L293 (-16.7985, -43.7616) -> (-16.3785, -43.9205)
  line L294 (-16.3785, -43.9205) -> (-15.1211, -42.5824)
  line L295 (-15.1211, -42.5824) -> (-14.0669, -41.1628)
  line L296 (-14.0669, -41.1628) -> (-12.8145, -41.5697)
  line L297 (-12.8145, -41.5697) -> (-12.7961, -43.3379)
  line L298 (-12.7961, -43.3379) -> (-12.5653, -45.1595)
  line L299 (-12.5653, -45.1595) -> (-12.1321, -45.2778)
  line L300 (-12.1321, -45.2778) -> (-11.6978, -45.3919)
  line L301 (-11.6978, -45.3919) -> (-10.5872, -43.9297)
  line L302 (-10.5872, -43.9297) -> (-9.6871, -42.4077)
  line L303 (-9.6871, -42.4077) -> (-8.3991, -42.6814)
  line L304 (-8.3991, -42.6814) -> (-8.196, -44.438)
  line L305 (-8.196, -44.438) -> (-7.7761, -46.2255)
  line L306 (-7.7761, -46.2255) -> (-7.3329, -46.2979)
  line L307 (-7.3329, -46.2979) -> (-6.889, -46.366)
  line L308 (-6.889, -46.366) -> (-5.9373, -44.7957)
  line L309 (-5.9373, -44.7957) -> (-5.2013, -43.1879)
  line L310 (-5.2013, -43.1879) -> (-3.8917, -43.3256)
  line L311 (-3.8917, -43.3256) -> (-3.506, -45.0513)
  line L312 (-3.506, -45.0513) -> (-2.9016, -46.7851)
  line L313 (-2.9016, -46.7851) -> (-2.4532, -46.8108)
  line L314 (-2.4532, -46.8108) -> (-2.0047, -46.8321)
  line L315 (-2.0047, -46.8321) -> (-1.2223, -45.171)
  line L316 (-1.2223, -45.171) -> (-0.6584, -43.495)
  line L317 (-0.6584, -43.495) -> (0.6584, -43.495)
  line L318 (0.6584, -43.495) -> (1.2223, -45.171)
  line L319 (1.2223, -45.171) -> (2.0047, -46.8321)
  line L320 (2.0047, -46.8321) -> (2.4532, -46.8108)
  line L321 (2.4532, -46.8108) -> (2.9016, -46.7851)
  line L322 (2.9016, -46.7851) -> (3.506, -45.0513)
  line L323 (3.506, -45.0513) -> (3.8917, -43.3256)
  line L324 (3.8917, -43.3256) -> (5.2013, -43.1879)
  line L325 (5.2013, -43.1879) -> (5.9373, -44.7957)
  line L326 (5.9373, -44.7957) -> (6.889, -46.366)
  line L327 (6.889, -46.366) -> (7.3329, -46.2979)
  line L328 (7.3329, -46.2979) -> (7.7761, -46.2255)
  line L329 (7.7761, -46.2255) -> (8.196, -44.438)
  line L330 (8.196, -44.438) -> (8.3991, -42.6814)
  line L331 (8.3991, -42.6814) -> (9.6871, -42.4077)
  line L332 (9.6871, -42.4077) -> (10.5872, -43.9297)
  line L333 (10.5872, -43.9297) -> (11.6978, -45.3919)
  line L334 (11.6978, -45.3919) -> (12.1321, -45.2778)
  line L335 (12.1321, -45.2778) -> (12.5653, -45.1595)
  line L336 (12.5653, -45.1595) -> (12.7961, -43.3379)
  line L337 (12.7961, -43.3379) -> (12.8145, -41.5697)
  line L338 (12.8145, -41.5697) -> (14.0669, -41.1628)
  line L339 (14.0669, -41.1628) -> (15.1211, -42.5824)
  line L340 (15.1211, -42.5824) -> (16.3785, -43.9205)
  line L341 (16.3785, -43.9205) -> (16.7985, -43.7616)
  line L342 (16.7985, -43.7616) -> (17.217, -43.5986)
  line L343 (17.217, -43.5986) -> (17.256, -41.7629)
  line L344 (17.256, -41.7629) -> (17.0895, -40.0025)
  line L345 (17.0895, -40.0025) -> (18.2925, -39.4669)
  line L346 (18.2925, -39.4669) -> (19.4893, -40.7686)
  line L347 (19.4893, -40.7686) -> (20.8797, -41.9679)
  line L348 (20.8797, -41.9679) -> (21.2808, -41.7659)
  line L349 (21.2808, -41.7659) -> (21.6799, -41.5601)
  line L350 (21.6799, -41.5601) -> (21.5269, -39.7304)
  line L351 (21.5269, -39.7304) -> (21.1773, -37.997)
  line L352 (21.1773, -37.997) -> (22.3177, -37.3386)
  line L353 (22.3177, -37.3386) -> (23.644, -38.508)
  line L354 (23.644, -38.508) -> (25.1522, -39.5555)
  line L355 (25.1522, -39.5555) -> (25.53, -39.3127)
  line L356 (25.53, -39.3127) -> (25.9054, -39.0663)
  line L357 (25.9054, -39.0663) -> (25.5619, -37.2625)
  line L358 (25.5619, -37.2625) -> (25.0331, -35.5752)
  line L359 (25.0331, -35.5752) -> (26.0984, -34.8012)
  line L360 (26.0984, -34.8012) -> (27.5397, -35.8256)
  line L361 (27.5397, -35.8256) -> (29.1491, -36.7096)
  line L362 (29.1491, -36.7096) -> (29.4994, -36.4287)
  line L363 (29.4994, -36.4287) -> (29.847, -36.1444)
  line L364 (29.847, -36.1444) -> (29.3169, -34.3865)
  line L365 (29.3169, -34.3865) -> (28.6146, -32.7636)
  line L366 (28.6146, -32.7636) -> (29.5931, -31.8825)
  line L367 (29.5931, -31.8825) -> (31.1336, -32.7507)
  line L368 (31.1336, -32.7507) -> (32.8266, -33.4616)
  line L369 (32.8266, -33.4616) -> (33.1456, -33.1456)
  line L370 (33.1456, -33.1456) -> (33.4616, -32.8266)
  line L371 (33.4616, -32.8266) -> (32.7507, -31.1336)
  line L372 (32.7507, -31.1336) -> (31.8825, -29.5931)
  line L373 (31.8825, -29.5931) -> (32.7636, -28.6146)
  line L374 (32.7636, -28.6146) -> (34.3865, -29.3169)
  line L375 (34.3865, -29.3169) -> (36.1444, -29.847)
  line L376 (36.1444, -29.847) -> (36.4287, -29.4994)
  line L377 (36.4287, -29.4994) -> (36.7096, -29.1491)
  line L378 (36.7096, -29.1491) -> (35.8256, -27.5397)
  line L379 (35.8256, -27.5397) -> (34.8012, -26.0984)
  line L380 (34.8012, -26.0984) -> (35.5752, -25.0331)
  line L381 (35.5752, -25.0331) -> (37.2625, -25.5619)
  line L382 (37.2625, -25.5619) -> (39.0663, -25.9054)
  line L383 (39.0663, -25.9054) -> (39.3127, -25.53)
  line L384 (39.3127, -25.53) -> (39.5555, -25.1522)
  line L385 (39.5555, -25.1522) -> (38.508, -23.644)
  line L386 (38.508, -23.644) -> (37.3386, -22.3177)
  line L387 (37.3386, -22.3177) -> (37.997, -21.1773)
  line L388 (37.997, -21.1773) -> (39.7304, -21.5269)
  line L389 (39.7304, -21.5269) -> (41.5601, -21.6799)
  line L390 (41.5601, -21.6799) -> (41.7659, -21.2808)
  line L391 (41.7659, -21.2808) -> (41.9679, -20.8797)
  line L392 (41.9679, -20.8797) -> (40.7686, -19.4893)
  line L393 (40.7686, -19.4893) -> (39.4669, -18.2925)
  line L394 (39.4669, -18.2925) -> (40.0025, -17.0895)
  line L395 (40.0025, -17.0895) -> (41.7629, -17.256)
  line L396 (41.7629, -17.256) -> (43.5986, -17.217)
  line L397 (43.5986, -17.217) -> (43.7616, -16.7985)
  line L398 (43.7616, -16.7985) -> (43.9205, -16.3785)
  line L399 (43.9205, -16.3785) -> (42.5824, -15.1211)
  line L400 (42.5824, -15.1211) -> (41.1628, -14.0669)
  line L401 (41.1628, -14.0669) -> (41.5697, -12.8145)
  line L402 (41.5697, -12.8145) -> (43.3379, -12.7961)
  line L403 (43.3379, -12.7961) -> (45.1595, -12.5653)
  line L404 (45.1595, -12.5653) -> (45.2778, -12.1321)
  line L405 (45.2778, -12.1321) -> (45.3919, -11.6978)
  line L406 (45.3919, -11.6978) -> (43.9297, -10.5872)
  line L407 (43.9297, -10.5872) -> (42.4077, -9.6871)
  line L408 (42.4077, -9.6871) -> (42.6814, -8.3991)
  line L409 (42.6814, -8.3991) -> (44.438, -8.196)
  line L410 (44.438, -8.196) -> (46.2255, -7.7761)
  line L411 (46.2255, -7.7761) -> (46.2979, -7.3329)
  line L412 (46.2979, -7.3329) -> (46.366, -6.889)
  line L413 (46.366, -6.889) -> (44.7957, -5.9373)
  line L414 (44.7957, -5.9373) -> (43.1879, -5.2013)
  line L415 (43.1879, -5.2013) -> (43.3256, -3.8917)
  line L416 (43.3256, -3.8917) -> (45.0513, -3.506)
  line L417 (45.0513, -3.506) -> (46.7851, -2.9016)
  line L418 (46.7851, -2.9016) -> (46.8108, -2.4532)
  line L419 (46.8108, -2.4532) -> (46.8321, -2.0047)
extrude "Stage2_Ring_Teeth_Cut" cut sketch "スケッチ3 (17)" along normal blind 15 from surface at 73 bodies 19 in component "Stage2_Internal_Ring_Gear"